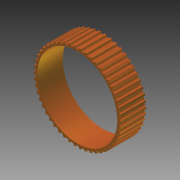
# Autodesk Inventor part: new wheel rim
Saved by Autodesk Inventor 2012 (Build 160160000, 160)
## iProperties
Created: 2012-08-10
Part Number: new wheel rim
Material: Default
Document SubType Name: Modeling
Designer: Bryce
Density: 1 g/cm^3
Author: Bryce
Autodesk Inventor part; units mm, degrees
ref_plane "YZ Plane" through (0, 0, 0) normal (1, 0, 0) x (0, 1, 0)
ref_plane "XZ Plane" through (0, 0, 0) normal (0, 1, 0) x (-1, 0, 0)
ref_plane "XY Plane" through (0, 0, 0) normal (0, 0, 1) x (1, 0, 0)
sketch "Sketch1" plane through (0, 0, 0) normal (0, 0, 1) x (1, 0, 0)
  circle A0 centre (0, 0) radius 34.925
  arc A1 (-1.5872, 38.0669) -> (0, 36.5125) centre (0, 38.1) ccw
  line L0 (0, 38.1) -> (0, 0) construction
  arc A2 (0, 36.5125) -> (1.5872, 38.0669) centre (0, 38.1) ccw
  arc A3 (-6.3457, 37.5678) -> (-4.5762, 36.2246) centre (-4.7752, 37.7996) ccw
  arc A4 (-4.5762, 36.2246) -> (-3.1964, 37.9657) centre (-4.7752, 37.7996) ccw
  arc A5 (-11.0042, 36.4763) -> (-9.0803, 35.3654) centre (-9.4751, 36.903) ccw
  arc A6 (-9.0803, 35.3654) -> (-7.9296, 37.2657) centre (-9.4751, 36.903) ccw
  arc A7 (-15.4891, 34.8095) -> (-13.4411, 33.9485) centre (-14.0255, 35.4245) ccw
  arc A8 (-13.4411, 33.9485) -> (-12.5377, 35.978) centre (-14.0255, 35.4245) ccw
  arc A9 (-19.7297, 32.5937) -> (-17.59, 31.9961) centre (-18.3548, 33.3873) ccw
  arc A10 (-17.59, 31.9961) -> (-16.948, 34.1229) centre (-18.3548, 33.3873) ccw
  arc A11 (-23.6592, 29.8639) -> (-21.4615, 29.5392) centre (-22.3946, 30.8235) ccw
  arc A12 (-21.4615, 29.5392) -> (-21.0911, 31.7297) centre (-22.3946, 30.8235) ccw
  arc A13 (-27.2156, 26.6631) -> (-24.9945, 26.6165) centre (-26.0812, 27.7737) ccw
  arc A14 (-24.9945, 26.6165) -> (-24.9016, 28.8361) centre (-26.0812, 27.7737) ccw
  arc A15 (-30.3428, 23.0418) -> (-28.1334, 23.2739) centre (-29.3566, 24.2859) ccw
  arc A16 (-28.1334, 23.2739) -> (-28.3194, 25.4877) centre (-29.3566, 24.2859) ccw
  arc A17 (-32.9914, 19.0572) -> (-30.8285, 19.5644) centre (-32.1689, 20.415) ccw
  arc A18 (-30.8285, 19.5644) -> (-31.2905, 21.7374) centre (-32.1689, 20.415) ccw
  arc A19 (-35.1198, 14.772) -> (-33.0375, 15.5463) centre (-34.4739, 16.2222) ccw
  arc A20 (-33.0375, 15.5463) -> (-33.7682, 17.6442) centre (-34.4739, 16.2222) ccw
  arc A21 (-36.6943, 10.2539) -> (-34.7255, 11.283) centre (-36.2353, 11.7735) ccw
  arc A22 (-34.7255, 11.283) -> (-35.7133, 13.2728) centre (-36.2353, 11.7735) ccw
  arc A23 (-37.6901, 5.574) -> (-35.8658, 6.8418) centre (-37.4251, 7.1392) ccw
  arc A24 (-35.8658, 6.8418) -> (-37.0953, 8.6921) centre (-37.4251, 7.1392) ccw
  arc A25 (-38.0915, 0.8062) -> (-36.4405, 2.2926) centre (-38.0248, 2.3923) ccw
  arc A26 (-36.4405, 2.2926) -> (-37.8922, 3.9743) centre (-38.0248, 2.3923) ccw
  arc A27 (-37.8922, -3.9743) -> (-36.4405, -2.2926) centre (-38.0248, -2.3923) ccw
  arc A28 (-36.4405, -2.2926) -> (-38.0915, -0.8062) centre (-38.0248, -2.3923) ccw
  arc A29 (-37.0953, -8.6921) -> (-35.8658, -6.8418) centre (-37.4251, -7.1392) ccw
  arc A30 (-35.8658, -6.8418) -> (-37.6901, -5.574) centre (-37.4251, -7.1392) ccw
  arc A31 (-35.7133, -13.2728) -> (-34.7255, -11.283) centre (-36.2353, -11.7735) ccw
  arc A32 (-34.7255, -11.283) -> (-36.6943, -10.2539) centre (-36.2353, -11.7735) ccw
  arc A33 (-33.7682, -17.6442) -> (-33.0375, -15.5463) centre (-34.4739, -16.2222) ccw
  arc A34 (-33.0375, -15.5463) -> (-35.1198, -14.772) centre (-34.4739, -16.2222) ccw
  arc A35 (-31.2905, -21.7374) -> (-30.8285, -19.5644) centre (-32.1689, -20.415) ccw
  arc A36 (-30.8285, -19.5644) -> (-32.9914, -19.0572) centre (-32.1689, -20.415) ccw
  arc A37 (-28.3194, -25.4877) -> (-28.1334, -23.2739) centre (-29.3566, -24.2859) ccw
  arc A38 (-28.1334, -23.2739) -> (-30.3428, -23.0418) centre (-29.3566, -24.2859) ccw
  arc A39 (-24.9016, -28.8361) -> (-24.9945, -26.6165) centre (-26.0812, -27.7737) ccw
  arc A40 (-24.9945, -26.6165) -> (-27.2156, -26.6631) centre (-26.0812, -27.7737) ccw
  arc A41 (-21.0911, -31.7297) -> (-21.4615, -29.5392) centre (-22.3946, -30.8235) ccw
  arc A42 (-21.4615, -29.5392) -> (-23.6592, -29.8639) centre (-22.3946, -30.8235) ccw
  arc A43 (-16.948, -34.1229) -> (-17.59, -31.9961) centre (-18.3548, -33.3873) ccw
  arc A44 (-17.59, -31.9961) -> (-19.7297, -32.5937) centre (-18.3548, -33.3873) ccw
  arc A45 (-12.5377, -35.978) -> (-13.4411, -33.9485) centre (-14.0255, -35.4245) ccw
  arc A46 (-13.4411, -33.9485) -> (-15.4891, -34.8095) centre (-14.0255, -35.4245) ccw
  arc A47 (-7.9296, -37.2657) -> (-9.0803, -35.3654) centre (-9.4751, -36.903) ccw
  arc A48 (-9.0803, -35.3654) -> (-11.0042, -36.4763) centre (-9.4751, -36.903) ccw
  arc A49 (-3.1964, -37.9657) -> (-4.5762, -36.2246) centre (-4.7752, -37.7996) ccw
  arc A50 (-4.5762, -36.2246) -> (-6.3457, -37.5678) centre (-4.7752, -37.7996) ccw
  arc A51 (1.5872, -38.0669) -> (0, -36.5125) centre (0, -38.1) ccw
  arc A52 (0, -36.5125) -> (-1.5872, -38.0669) centre (0, -38.1) ccw
  arc A53 (6.3457, -37.5678) -> (4.5762, -36.2246) centre (4.7752, -37.7996) ccw
  arc A54 (4.5762, -36.2246) -> (3.1964, -37.9657) centre (4.7752, -37.7996) ccw
  arc A55 (11.0042, -36.4763) -> (9.0803, -35.3654) centre (9.4751, -36.903) ccw
  arc A56 (9.0803, -35.3654) -> (7.9296, -37.2657) centre (9.4751, -36.903) ccw
  arc A57 (15.4891, -34.8095) -> (13.4411, -33.9485) centre (14.0255, -35.4245) ccw
  arc A58 (13.4411, -33.9485) -> (12.5377, -35.978) centre (14.0255, -35.4245) ccw
  arc A59 (19.7297, -32.5937) -> (17.59, -31.9961) centre (18.3548, -33.3873) ccw
  arc A60 (17.59, -31.9961) -> (16.948, -34.1229) centre (18.3548, -33.3873) ccw
  arc A61 (23.6592, -29.8639) -> (21.4615, -29.5392) centre (22.3946, -30.8235) ccw
  arc A62 (21.4615, -29.5392) -> (21.0911, -31.7297) centre (22.3946, -30.8235) ccw
  arc A63 (27.2156, -26.6631) -> (24.9945, -26.6165) centre (26.0812, -27.7737) ccw
  arc A64 (24.9945, -26.6165) -> (24.9016, -28.8361) centre (26.0812, -27.7737) ccw
  arc A65 (30.3428, -23.0418) -> (28.1334, -23.2739) centre (29.3566, -24.2859) ccw
  arc A66 (28.1334, -23.2739) -> (28.3194, -25.4877) centre (29.3566, -24.2859) ccw
  arc A67 (32.9914, -19.0572) -> (30.8285, -19.5644) centre (32.1689, -20.415) ccw
  arc A68 (30.8285, -19.5644) -> (31.2905, -21.7374) centre (32.1689, -20.415) ccw
  arc A69 (35.1198, -14.772) -> (33.0375, -15.5463) centre (34.4739, -16.2222) ccw
  arc A70 (33.0375, -15.5463) -> (33.7682, -17.6442) centre (34.4739, -16.2222) ccw
  arc A71 (-11.0042, 36.4763) -> (-12.5377, 35.978) centre (0, 0) ccw
  arc A72 (-7.9296, 37.2657) -> (-11.0042, 36.4763) centre (0, 0) ccw construction
  arc A73 (-6.3457, 37.5678) -> (-7.9296, 37.2657) centre (0, 0) ccw
  arc A74 (-3.1964, 37.9657) -> (-6.3457, 37.5678) centre (0, 0) ccw construction
  arc A75 (-12.5377, 35.978) -> (-15.4891, 34.8095) centre (0, 0) ccw construction
  arc A76 (-15.4891, 34.8095) -> (-16.948, 34.1229) centre (0, 0) ccw
  arc A77 (-16.948, 34.1229) -> (-19.7297, 32.5937) centre (0, 0) ccw construction
  arc A78 (-19.7297, 32.5937) -> (-21.0911, 31.7297) centre (0, 0) ccw
  arc A79 (-21.0911, 31.7297) -> (-23.6592, 29.8639) centre (0, 0) ccw construction
  arc A80 (-23.6592, 29.8639) -> (-24.9016, 28.8361) centre (0, 0) ccw
  arc A81 (-27.2156, 26.6631) -> (-28.3194, 25.4877) centre (0, 0) ccw
  arc A82 (-28.3194, 25.4877) -> (-30.3428, 23.0418) centre (0, 0) ccw construction
  arc A83 (-30.3428, 23.0418) -> (-31.2905, 21.7374) centre (0, 0) ccw
  arc A84 (-32.9914, 19.0572) -> (-33.7682, 17.6442) centre (0, 0) ccw
  arc A85 (-31.2905, 21.7374) -> (-32.9914, 19.0572) centre (0, 0) ccw construction
  arc A86 (-33.7682, 17.6442) -> (-35.1198, 14.772) centre (0, 0) ccw construction
  arc A87 (-35.1198, 14.772) -> (-35.7133, 13.2728) centre (0, 0) ccw
  arc A88 (-24.9016, 28.8361) -> (-27.2156, 26.6631) centre (0, 0) ccw construction
  arc A89 (-36.6943, 10.2539) -> (-37.0953, 8.6921) centre (0, 0) ccw
  arc A90 (-37.6901, 5.574) -> (-37.8922, 3.9743) centre (0, 0) ccw
  arc A91 (-38.0915, 0.8062) -> (-38.0915, -0.8062) centre (0, 0) ccw
  arc A92 (-37.8922, 3.9743) -> (-38.0915, 0.8062) centre (0, 0) ccw construction
  arc A93 (-37.0953, 8.6921) -> (-37.6901, 5.574) centre (0, 0) ccw construction
  arc A94 (-35.7133, 13.2728) -> (-36.6943, 10.2539) centre (0, 0) ccw construction
  arc A95 (-38.0915, -0.8062) -> (-37.8922, -3.9743) centre (0, 0) ccw construction
  arc A96 (-37.8922, -3.9743) -> (-37.6901, -5.574) centre (0, 0) ccw
  arc A97 (-37.6901, -5.574) -> (-37.0953, -8.6921) centre (0, 0) ccw construction
  arc A98 (-37.0953, -8.6921) -> (-36.6943, -10.2539) centre (0, 0) ccw
  arc A99 (-36.6943, -10.2539) -> (-35.7133, -13.2728) centre (0, 0) ccw construction
  arc A100 (-35.7133, -13.2728) -> (-35.1198, -14.772) centre (0, 0) ccw
  arc A101 (-35.1198, -14.772) -> (-33.7682, -17.6442) centre (0, 0) ccw construction
  arc A102 (-33.7682, -17.6442) -> (-32.9914, -19.0572) centre (0, 0) ccw
  arc A103 (-32.9914, -19.0572) -> (-31.2905, -21.7374) centre (0, 0) ccw construction
  arc A104 (-31.2905, -21.7374) -> (-30.3428, -23.0418) centre (0, 0) ccw
  arc A105 (-28.3194, -25.4877) -> (-27.2156, -26.6631) centre (0, 0) ccw
  arc A106 (-27.2156, -26.6631) -> (-24.9016, -28.8361) centre (0, 0) ccw construction
  arc A107 (-24.9016, -28.8361) -> (-23.6592, -29.8639) centre (0, 0) ccw
  arc A108 (-23.6592, -29.8639) -> (-21.0911, -31.7297) centre (0, 0) ccw construction
  arc A109 (-21.0911, -31.7297) -> (-19.7297, -32.5937) centre (0, 0) ccw
  arc A110 (-19.7297, -32.5937) -> (-16.948, -34.1229) centre (0, 0) ccw construction
  arc A111 (-16.948, -34.1229) -> (-15.4891, -34.8095) centre (0, 0) ccw
  arc A112 (-15.4891, -34.8095) -> (-12.5377, -35.978) centre (0, 0) ccw construction
  arc A113 (-12.5377, -35.978) -> (-11.0042, -36.4763) centre (0, 0) ccw
  arc A114 (-11.0042, -36.4763) -> (-7.9296, -37.2657) centre (0, 0) ccw construction
  arc A115 (-7.9296, -37.2657) -> (-6.3457, -37.5678) centre (0, 0) ccw
  arc A116 (-6.3457, -37.5678) -> (-3.1964, -37.9657) centre (0, 0) ccw construction
  arc A117 (-3.1964, -37.9657) -> (-1.5872, -38.0669) centre (0, 0) ccw
  arc A118 (-1.5872, -38.0669) -> (1.5872, -38.0669) centre (0, 0) ccw construction
  arc A119 (1.5872, -38.0669) -> (3.1964, -37.9657) centre (0, 0) ccw
  arc A120 (3.1964, -37.9657) -> (6.3457, -37.5678) centre (0, 0) ccw construction
  arc A121 (6.3457, -37.5678) -> (7.9296, -37.2657) centre (0, 0) ccw
  arc A122 (-30.3428, -23.0418) -> (-28.3194, -25.4877) centre (0, 0) ccw construction
  arc A123 (7.9296, -37.2657) -> (11.0042, -36.4763) centre (0, 0) ccw construction
  arc A124 (11.0042, -36.4763) -> (12.5377, -35.978) centre (0, 0) ccw
  arc A125 (12.5377, -35.978) -> (15.4891, -34.8095) centre (0, 0) ccw construction
  arc A126 (16.948, -34.1229) -> (19.7297, -32.5937) centre (0, 0) ccw construction
  arc A127 (19.7297, -32.5937) -> (21.0911, -31.7297) centre (0, 0) ccw
  arc A128 (15.4891, -34.8095) -> (16.948, -34.1229) centre (0, 0) ccw
  arc A129 (23.6592, -29.8639) -> (24.9016, -28.8361) centre (0, 0) ccw
  arc A130 (21.0911, -31.7297) -> (23.6592, -29.8639) centre (0, 0) ccw construction
  arc A131 (24.9016, -28.8361) -> (27.2156, -26.6631) centre (0, 0) ccw construction
  arc A132 (27.2156, -26.6631) -> (28.3194, -25.4877) centre (0, 0) ccw
  arc A133 (28.3194, -25.4877) -> (30.3428, -23.0418) centre (0, 0) ccw construction
  arc A134 (30.3428, -23.0418) -> (31.2905, -21.7374) centre (0, 0) ccw
  arc A135 (31.2905, -21.7374) -> (32.9914, -19.0572) centre (0, 0) ccw construction
  arc A136 (32.9914, -19.0572) -> (33.7682, -17.6442) centre (0, 0) ccw
  arc A137 (33.7682, -17.6442) -> (35.1198, -14.772) centre (0, 0) ccw construction
  arc A138 (1.5872, 38.0669) -> (0, 38.1) centre (0, 0) ccw construction
  arc A139 (0, 38.1) -> (-1.5872, 38.0669) centre (0, 0) ccw construction
  arc A140 (-1.5872, 38.0669) -> (-3.1964, 37.9657) centre (0, 0) ccw
  arc A141 (36.6943, -10.2539) -> (34.7255, -11.283) centre (36.2353, -11.7735) ccw
  arc A142 (34.7255, -11.283) -> (35.7133, -13.2728) centre (36.2353, -11.7735) ccw
  arc A143 (37.6901, -5.574) -> (35.8658, -6.8418) centre (37.4251, -7.1392) ccw
  arc A144 (35.8658, -6.8418) -> (37.0953, -8.6921) centre (37.4251, -7.1392) ccw
  arc A145 (38.0915, -0.8062) -> (36.4405, -2.2926) centre (38.0248, -2.3923) ccw
  arc A146 (36.4405, -2.2926) -> (37.8922, -3.9743) centre (38.0248, -2.3923) ccw
  arc A147 (37.8922, 3.9743) -> (36.4405, 2.2926) centre (38.0248, 2.3923) ccw
  arc A148 (36.4405, 2.2926) -> (38.0915, 0.8062) centre (38.0248, 2.3923) ccw
  arc A149 (37.0953, 8.6921) -> (35.8658, 6.8418) centre (37.4251, 7.1392) ccw
  arc A150 (35.8658, 6.8418) -> (37.6901, 5.574) centre (37.4251, 7.1392) ccw
  arc A151 (35.7133, 13.2728) -> (34.7255, 11.283) centre (36.2353, 11.7735) ccw
  arc A152 (34.7255, 11.283) -> (36.6943, 10.2539) centre (36.2353, 11.7735) ccw
  arc A153 (33.7682, 17.6442) -> (33.0375, 15.5463) centre (34.4739, 16.2222) ccw
  arc A154 (33.0375, 15.5463) -> (35.1198, 14.772) centre (34.4739, 16.2222) ccw
  arc A155 (31.2905, 21.7374) -> (30.8285, 19.5644) centre (32.1689, 20.415) ccw
  arc A156 (30.8285, 19.5644) -> (32.9914, 19.0572) centre (32.1689, 20.415) ccw
  arc A157 (28.3194, 25.4877) -> (28.1334, 23.2739) centre (29.3566, 24.2859) ccw
  arc A158 (28.1334, 23.2739) -> (30.3428, 23.0418) centre (29.3566, 24.2859) ccw
  arc A159 (24.9016, 28.8361) -> (24.9945, 26.6165) centre (26.0812, 27.7737) ccw
  arc A160 (24.9945, 26.6165) -> (27.2156, 26.6631) centre (26.0812, 27.7737) ccw
  arc A161 (21.0911, 31.7297) -> (21.4615, 29.5392) centre (22.3946, 30.8235) ccw
  arc A162 (21.4615, 29.5392) -> (23.6592, 29.8639) centre (22.3946, 30.8235) ccw
  arc A163 (16.948, 34.1229) -> (17.59, 31.9961) centre (18.3548, 33.3873) ccw
  arc A164 (17.59, 31.9961) -> (19.7297, 32.5937) centre (18.3548, 33.3873) ccw
  arc A165 (12.5377, 35.978) -> (13.4411, 33.9485) centre (14.0255, 35.4245) ccw
  arc A166 (13.4411, 33.9485) -> (15.4891, 34.8095) centre (14.0255, 35.4245) ccw
  arc A167 (7.9296, 37.2657) -> (9.0803, 35.3654) centre (9.4751, 36.903) ccw
  arc A168 (9.0803, 35.3654) -> (11.0042, 36.4763) centre (9.4751, 36.903) ccw
  arc A169 (3.1964, 37.9657) -> (4.5762, 36.2246) centre (4.7752, 37.7996) ccw
  arc A170 (4.5762, 36.2246) -> (6.3457, 37.5678) centre (4.7752, 37.7996) ccw
  arc A171 (3.1964, 37.9657) -> (1.5872, 38.0669) centre (0, 0) ccw
  arc A172 (7.9296, 37.2657) -> (6.3457, 37.5678) centre (0, 0) ccw
  arc A173 (12.5377, 35.978) -> (11.0042, 36.4763) centre (0, 0) ccw
  arc A174 (16.948, 34.1229) -> (15.4891, 34.8095) centre (0, 0) ccw
  arc A175 (21.0911, 31.7297) -> (19.7297, 32.5937) centre (0, 0) ccw
  arc A176 (24.9016, 28.8361) -> (23.6592, 29.8639) centre (0, 0) ccw
  arc A177 (28.3194, 25.4877) -> (27.2156, 26.6631) centre (0, 0) ccw
  arc A178 (31.2905, 21.7374) -> (30.3428, 23.0418) centre (0, 0) ccw
  arc A179 (33.7682, 17.6442) -> (32.9914, 19.0572) centre (0, 0) ccw
  arc A180 (35.7133, 13.2728) -> (35.1198, 14.772) centre (0, 0) ccw
  arc A181 (37.0953, 8.6921) -> (36.6943, 10.2539) centre (0, 0) ccw
  arc A182 (37.8922, 3.9743) -> (37.6901, 5.574) centre (0, 0) ccw
  arc A183 (38.0915, -0.8062) -> (38.0915, 0.8062) centre (0, 0) ccw
  arc A184 (37.6901, -5.574) -> (37.8922, -3.9743) centre (0, 0) ccw
  arc A185 (35.1198, -14.772) -> (35.7133, -13.2728) centre (0, 0) ccw
  arc A186 (36.6943, -10.2539) -> (37.0953, -8.6921) centre (0, 0) ccw
  dimension "d10" = 76.2
  dimension "d0" = 69.85
  dimension "d1" = 38.1
  dimension "d5" = 360
  dimension "d17" = 1.5875
  constraints: 198 point on circle, 100 centre point, 4 vertical alignment, 2 end point, 2 point on line, 1 coincident, 1 horizontal alignment, 1 line through centre, 1 vertical, 558 other
  measures "d0" diameter of A0
  measures "d1" distance of point (0, 0) L0.start
  measures "d17" radius of A2
extrude "Extrusion1" add sketch "Sketch1" along normal blind 22.225
body "Solid1"
